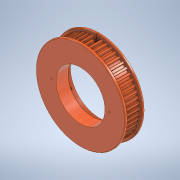
# Autodesk Inventor part: 004
Saved by Autodesk Inventor 2020 (Build 240168000, 168)
## iProperties
Created: 2024-01-30
Part Number: 004
Material: PBT Plastic
Document SubType Name: Modeling
Designer: Scott Bricker
Density: 1.31 g/cm^3
Appearance: Smooth - Light Orange
Mass: 116.199 g
Surface Area: 268.297 cm^2
Volume: 88.7017 cm^3
Project: Motorized Rotator Mount
Description: Output Gear Actuator
Engineer: Scott Bricker
Author: Scott Bricker
Title: Output Gear Actuator
Revision Number: v2.2
Comments: This part slides onto and is fixed to a rotational component which is fixed in space.
Autodesk Inventor part; units mm, degrees
ref_plane "YZ Plane" through (0, 0, 0) normal (1, 0, 0) x (0, 1, 0)
sketch "Sketch1" plane through (0, 0, 0) normal (0, 0, 1) x (1, 0, 0)
  circle A0 centre (0, 0) radius 50
  dimension "d0" = 100
  constraints: 1 centre point, 1 coincident
  measures "d0" diameter of A0
extrude "Extrusion1" add sketch "Sketch1" along normal blind 2
sketch "Sketch2" plane through (0, 0, 2) normal (0, 0, 1) x (1, 0, 0)
  circle A0 centre (0, 0) radius 45
  dimension "d3" = 90
  constraints: 1 centre point, 1 coincident
  measures "d3" diameter of A0
extrude "Extrusion2" add sketch "Sketch2" along normal blind 16.5
sketch "Sketch3" plane through (0, 0, 2) normal (0, 0, 1) x (1, 0, 0)
  circle A0 centre (0, 0) radius 45 projected
  circle A1 centre (0, 0) radius 50 projected
  circle A2 centre (0, 0) radius 45 projected
  line L0 (0, 0) -> (0, 60.687)
  line L1 (0, 0) -> (-1.2885, 46.7446)
  line L2 (0, 0) -> (1.2885, 46.7446)
  circle A3 centre (0, 0) radius 47.1736
  line L3 (-0.8886, 47.1556) -> (0.8886, 47.1556)
  arc A4 (-0.8886, 47.1556) -> (-1.2885, 46.7446) centre (-0.8886, 46.7556) ccw
  arc A5 (1.2885, 46.7446) -> (0.8886, 47.1556) centre (0.8886, 46.7556) ccw
  point P0 (-1.2998, 47.1556)
  point P1 (1.2998, 47.1556)
  point P2 (-1.2399, 44.9829)
  point P3 (1.2399, 44.9829)
  dimension "d6" = 94.3471
  dimension "d7" = 1.579
  dimension "d8" = 1.579
  dimension "d9" = 0.4
  dimension "d10" = 0.4
  constraints: 8 end point, 6 point on circle, 4 point on line, 4 tangent, 3 centre point, 1 coincident, 1 vertical
  measures "d6" diameter of A3
  measures "d7" angle of L0 L1
  measures "d8" angle of L0 L2
  measures "d9" radius of A4
  measures "d10" radius of A5
extrude "Extrusion3" add sketch "Sketch3" along normal blind 16 contours A0 L0 L3 A5 L2 | L1 A4 L3 L0 A0
pattern_circular "Circular Pattern1" count 57 over 360 about axis through (0, 0, 2) along (0, 0, 1) of "Extrusion3"
sketch "Sketch4" plane through (0, 0, 18.5) normal (0, 0, 1) x (1, 0, 0)
  circle A0 centre (0, 0) radius 50
  dimension "d16" = 100
  constraints: 1 centre point, 1 coincident
  measures "d16" diameter of A0
extrude "Extrusion4" add sketch "Sketch4" along normal blind 2
sketch "Sketch5" plane through (0, 0, 20.5) normal (0, 0, 1) x (1, 0, 0)
  circle A0 centre (0, 0) radius 50
  dimension "d19" = 100
  constraints: 1 centre point, 1 coincident
  measures "d19" diameter of A0
extrude "Extrusion5" add sketch "Sketch5" along normal blind 0.9
sketch "Sketch6" plane through (0, 0, 21.4) normal (0, 0, 1) x (1, 0, 0)
  circle A0 centre (0, 0) radius 32.5
  circle A1 centre (-32.5, 0) radius 0.5
  circle A2 centre (32.5, 0) radius 0.5
  dimension "d22" = 65
  dimension "d23" = 1
  dimension "d24" = 1
  constraints: 3 centre point, 2 point on circle, 1 coincident
  measures "d22" diameter of A0
  measures "d23" diameter of A1
  measures "d24" diameter of A2
extrude "Extrusion6" cut sketch "Sketch6" against normal blind 10 contours A0 A2 | A0 A2 | A1 A0 | A0 A1
sketch "Sketch7" plane through (0, 0, 0) normal (0, 0, -1) x (-1, 0, 0)
  circle A0 centre (0, 0) radius 32.8
  dimension "d27" = 65.6
  constraints: 1 centre point, 1 coincident
  measures "d27" diameter of A0
extrude "Extrusion7" cut sketch "Sketch7" against normal blind 7.9
sketch "Sketch8" plane through (0, 0, 7.9) normal (0, 0, -1) x (-1, 0, 0)
  circle A0 centre (0, 0) radius 27.5
  dimension "d30" = 55
  constraints: 1 centre point, 1 coincident
  measures "d30" diameter of A0
extrude "Extrusion8" cut sketch "Sketch8" against normal blind 50
ref_plane "Work Plane1" through (0, 47.75, 0) normal (0, 1, 0) x (-1, 0, 0)
sketch "Sketch9" plane through (0, 47.75, 0) normal (0, 1, 0) x (-1, 0, 0)
  line L0 (50, 21.4) -> (-50, 21.4) projected
  line L1 (50, 18.5) -> (-50, 18.5) projected
  line L2 (50, 2) -> (-50, 2) projected
  line L3 (50, 0) -> (-50, 0) projected
  line L4 (0.8886, 2) -> (-0.8886, 2) projected
  line L5 (0.8886, 2) -> (0.8886, 18) projected
  line L6 (-0.8886, 2) -> (-0.8886, 18) projected
  line L7 (50, 18.5) -> (-50, 18.5) projected
  line L8 (0.8886, 2) -> (-0.8886, 2) projected
  circle A0 centre (0, 4.1) radius 1.25
  line L9 (-0.8886, 18) -> (0.8886, 18) projected
  point P0 (0, 0)
  point P1 (0.8886, 18)
  dimension "d35" = 2.5
  dimension "d36" = 2.1
  constraints: 1 centre point, 1 other
  measures "d35" diameter of A0
  measures "d36" distance from line of L2 A0.centre
extrude "Extrusion9" cut sketch "Sketch9" against normal blind 50 contours A0 L6 L5 | L5 A0 | A0 L6
ref_plane "Work Plane2" through (0, -47.75, 0) normal (0, 1, 0) x (-1, 0, 0)
sketch "Sketch12" plane through (-0.8886, 47.1556, 2) normal (0, 1, 0) x (1, 0, 0)
  arc A0 (1.7772, -1.2209) -> (0, -1.2209) centre (0.8886, -2.1) ccw projected
  circle A1 centre (0.8886, -2.1) radius 2.625
  point P0 (0.8886, 2)
  dimension "d47" = 5.25
  constraints: 1 centre point, 1 coincident
  measures "d47" diameter of A1
extrude "Extrusion12" cut sketch "Sketch12" against normal mid plane 10
pattern_circular "Circular Pattern2" count 3 over 360 about axis through (0, 0, 18.5) along (0, 0, 1) of "Extrusion12", "Extrusion9"
fillet "Fillet1" radius 0.5 39 edges at (-50, 0, 18.5) (0, -50, 2) (35.9079, 34.794, 2) (48.4941, -12.1786, 2) (-43.3013, 25, 2) (-50, 0, 21.4) (-1.1776, 47.0322, 6.446) (-1.2643, 45.8663, 6.4005) (0, 47.1556, 6.725) (1.2643, 45.8663, 6.4005) (1.1776, 47.0322, 6.446) (2.3718, 44.9375, 2.9751) (2.2956, 44.9414, 5.3731) (-2.6203, 44.9236, 4.2568) (-1.575, 47.4738, 2) (1.575, 47.4738, 2) (-0.0055, 50, 1.475) (40.2152, -20.1926, 4.2568) (41.901, -22.3729, 2) (40.326, -25.1009, 2) (43.3037, -24.9958, 1.475) (37.7311, -24.5227, 2.9751) (37.7726, -24.4587, 5.3731) (41.3199, -22.4962, 6.446) (40.3535, -21.8383, 6.4005) (40.1422, -24.5359, 6.446) (39.0893, -24.028, 6.4005) (40.838, -23.5778, 6.725) (-37.5949, -24.7311, 4.2568) (-40.326, -25.1009, 2) (-43.2988, -25.0042, 1.475) (-41.901, -22.3729, 2) (-40.1029, -20.4147, 2.9751) (-40.0682, -20.4827, 5.3731) (-40.1422, -24.5359, 6.446) (-39.0893, -24.028, 6.4005) (-41.3199, -22.4962, 6.446) (-40.3535, -21.8383, 6.4005) (-40.838, -23.5778, 6.725)
body "Solid1"
